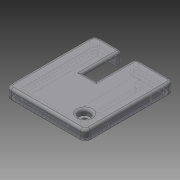
# Autodesk Inventor part: CaseTop_V3
Saved by Autodesk Inventor 2015 SP2 (Build 190223200, 223)
## iProperties
Created: 2016-03-02
Part Number: CaseTop_V3
Material: Generic
Document SubType Name: Modeling
Designer: Iain
Density: 1 g/cm^3
Appearance: Default
Author: Iain
Autodesk Inventor part; units mm, degrees
ref_plane "YZ Plane" through (0, 0, 0) normal (1, 0, 0) x (0, 1, 0)
ref_plane "XZ Plane" through (0, 0, 0) normal (0, 1, 0) x (-1, 0, 0)
ref_plane "XY Plane" through (0, 0, 0) normal (0, 0, 1) x (1, 0, 0)
sketch "Sketch1" plane through (0, 0, 0) normal (0, 0, 1) x (1, 0, 0)
  line L0 (20.25, -0.0291) -> (-20.25, -0.0291) construction
  arc A0 (-20.25, -0.0291) -> (-36.25, -16.0291) centre (-20.25, -16.0291) ccw construction
  line L1 (-36.25, -16.0291) -> (-36.25, -62.0291) construction
  arc A1 (-36.25, -62.0291) -> (-20.25, -78.0291) centre (-20.25, -62.0291) ccw construction
  line L2 (-20.25, -78.0291) -> (20.25, -78.0291) construction
  arc A2 (20.25, -78.0291) -> (36.25, -62.0291) centre (20.25, -62.0291) ccw construction
  line L3 (36.25, -62.0291) -> (36.25, -16.0291) construction
  arc A3 (36.25, -16.0291) -> (20.25, -0.0291) centre (20.25, -16.0291) ccw construction
  circle A4 centre (-34.25, -18.0291) radius 0.5 construction
  circle A5 centre (-34.25, -24.0291) radius 0.5 construction
  circle A6 centre (-34.25, -30.0291) radius 0.5 construction
  circle A7 centre (-34.25, -36.0291) radius 0.5 construction
  circle A8 centre (-34.25, -57.0291) radius 0.5 construction
  circle A9 centre (-34.25, -51.0291) radius 0.5 construction
  circle A10 centre (-34.25, -45.0291) radius 0.5 construction
  circle A11 centre (-34.25, -39.0291) radius 0.5 construction
  circle A12 centre (-34.25, -42.0291) radius 0.5 construction
  circle A13 centre (-34.25, -48.0291) radius 0.5 construction
  circle A14 centre (-34.25, -54.0291) radius 0.5 construction
  circle A15 centre (-34.25, -60.0291) radius 0.5 construction
  circle A16 centre (-34.25, -33.0291) radius 0.5 construction
  circle A17 centre (-34.25, -27.0291) radius 0.5 construction
  circle A18 centre (-34.25, -21.0291) radius 0.5 construction
  circle A19 centre (34.25, -27.0291) radius 0.5 construction
  circle A20 centre (34.25, -33.0291) radius 0.5 construction
  circle A21 centre (34.25, -60.0291) radius 0.5 construction
  circle A22 centre (34.25, -54.0291) radius 0.5 construction
  circle A23 centre (34.25, -48.0291) radius 0.5 construction
  circle A24 centre (34.25, -42.0291) radius 0.5 construction
  circle A25 centre (34.25, -39.0291) radius 0.5 construction
  circle A26 centre (34.25, -45.0291) radius 0.5 construction
  circle A27 centre (34.25, -51.0291) radius 0.5 construction
  circle A28 centre (34.25, -57.0291) radius 0.5 construction
  circle A29 centre (34.25, -36.0291) radius 0.5 construction
  circle A30 centre (34.25, -30.0291) radius 0.5 construction
  circle A31 centre (34.25, -24.0291) radius 0.5 construction
  circle A32 centre (34.25, -18.0291) radius 0.5 construction
  circle A33 centre (34.25, -21.0291) radius 0.5 construction
  circle A34 centre (-18, -76.0291) radius 0.5 construction
  circle A35 centre (-12, -76.0291) radius 0.5 construction
  circle A36 centre (-6, -76.0291) radius 0.5 construction
  circle A37 centre (18, -76.0291) radius 0.5 construction
  circle A38 centre (12, -76.0291) radius 0.5 construction
  circle A39 centre (6, -76.0291) radius 0.5 construction
  circle A40 centre (0, -76.0291) radius 0.5 construction
  circle A41 centre (3, -76.0291) radius 0.5 construction
  circle A42 centre (9, -76.0291) radius 0.5 construction
  circle A43 centre (15, -76.0291) radius 0.5 construction
  circle A44 centre (-3, -76.0291) radius 0.5 construction
  circle A45 centre (-9, -76.0291) radius 0.5 construction
  circle A46 centre (-15, -76.0291) radius 0.5 construction
  circle A47 centre (-9, -2.0291) radius 0.5 construction
  circle A48 centre (-3, -2.0291) radius 0.5 construction
  circle A49 centre (15, -2.0291) radius 0.5 construction
  circle A50 centre (9, -2.0291) radius 0.5 construction
  circle A51 centre (3, -2.0291) radius 0.5 construction
  circle A52 centre (0, -2.0291) radius 0.5 construction
  circle A53 centre (6, -2.0291) radius 0.5 construction
  circle A54 centre (12, -2.0291) radius 0.5 construction
  circle A55 centre (18, -2.0291) radius 0.5 construction
  circle A56 centre (-6, -2.0291) radius 0.5 construction
  circle A57 centre (-12, -2.0291) radius 0.5 construction
  circle A58 centre (-18, -2.0291) radius 0.5 construction
  circle A59 centre (-15, -2.0291) radius 0.5 construction
  arc A60 (-24.75, -62.0291) -> (-20.25, -66.5291) centre (-20.25, -62.0291) ccw construction
  line L4 (-24.75, -16.0291) -> (-24.75, -62.0291) construction
  arc A61 (-20.25, -11.5291) -> (-24.75, -16.0291) centre (-20.25, -16.0291) ccw construction
  line L5 (20.25, -11.5291) -> (-20.25, -11.5291) construction
  arc A62 (24.75, -16.0291) -> (20.25, -11.5291) centre (20.25, -16.0291) ccw construction
  line L6 (24.75, -62.0291) -> (24.75, -16.0291) construction
  arc A63 (20.25, -66.5291) -> (24.75, -62.0291) centre (20.25, -62.0291) ccw construction
  line L7 (-20.25, -66.5291) -> (20.25, -66.5291) construction
  line L8 (-20.25, -15.2291) -> (7.75, -15.2291) construction
  arc A64 (-20.25, -15.2291) -> (-21.05, -16.0291) centre (-20.25, -16.0291) ccw construction
  line L9 (-21.05, -62.0291) -> (-21.05, -16.0291) construction
  arc A65 (-21.05, -62.0291) -> (-20.25, -62.8291) centre (-20.25, -62.0291) ccw construction
  line L10 (20.25, -62.8291) -> (-20.25, -62.8291) construction
  arc A66 (20.25, -62.8291) -> (21.05, -62.0291) centre (20.25, -62.0291) ccw construction
  line L11 (21.05, -23.4291) -> (21.05, -62.0291) construction
  line L12 (21.05, -23.4291) -> (20.25, -23.4291) construction
  line L13 (20.25, -23.4291) -> (20.25, -48.5291) projected
  line L14 (20.25, -48.5291) -> (11.35, -48.5291) projected
  line L15 (11.35, -48.5291) -> (11.35, -23.4291) projected
  line L16 (11.35, -23.4291) -> (11.25, -23.4291) construction
  line L17 (11.25, -23.4291) -> (11.25, -19.4291) construction
  line L18 (11.25, -19.4291) -> (10.25, -19.4291) construction
  line L19 (10.25, -48.5291) -> (10.25, -19.4291) construction
  arc A67 (10.25, -48.5291) -> (11.25, -49.5291) centre (11.25, -48.5291) ccw construction
  line L20 (19.45, -49.5291) -> (11.25, -49.5291) construction
  line L21 (19.45, -62.5291) -> (19.45, -49.5291) construction
  line L22 (-20.75, -62.5291) -> (19.45, -62.5291) construction
  line L23 (-20.75, -15.5291) -> (-20.75, -62.5291) construction
  line L24 (7.75, -15.5291) -> (-20.75, -15.5291) construction
  line L25 (7.75, -15.5291) -> (7.75, -15.2291) construction
  line L26 (21.85, -16.0291) -> (21.85, -62.0291) projected
  arc A68 (20.25, -63.6291) -> (21.85, -62.0291) centre (20.25, -62.0291) ccw projected
  line L27 (20.25, -63.6291) -> (-20.25, -63.6291) projected
  arc A69 (-21.85, -62.0291) -> (-20.25, -63.6291) centre (-20.25, -62.0291) ccw projected
  line L28 (-21.85, -62.0291) -> (-21.85, -16.0291) projected
  arc A70 (-20.25, -14.4291) -> (-21.85, -16.0291) centre (-20.25, -16.0291) ccw projected
  line L29 (-20.25, -14.4291) -> (20.25, -14.4291) projected
  arc A71 (21.85, -16.0291) -> (20.25, -14.4291) centre (20.25, -16.0291) ccw projected
  arc A72 (20.25, -65.0291) -> (23.25, -62.0291) centre (20.25, -62.0291) ccw projected
  line L30 (23.25, -62.0291) -> (23.25, -16.0291) projected
  arc A73 (23.25, -16.0291) -> (20.25, -13.0291) centre (20.25, -16.0291) ccw projected
  line L31 (20.25, -13.0291) -> (-20.25, -13.0291) projected
  arc A74 (-20.25, -13.0291) -> (-23.25, -16.0291) centre (-20.25, -16.0291) ccw projected
  line L32 (-23.25, -16.0291) -> (-23.25, -62.0291) projected
  arc A75 (-23.25, -62.0291) -> (-20.25, -65.0291) centre (-20.25, -62.0291) ccw projected
  line L33 (-20.25, -65.0291) -> (20.25, -65.0291) projected
  line L34 (-8.75, -17.5291) -> (-2.25, -17.5291) construction
  arc A76 (-0.75, -16.0291) -> (-2.25, -17.5291) centre (-0.75, -17.5291) ccw construction
  line L35 (-10.25, -16.0291) -> (-0.75, -16.0291) projected
  arc A77 (-8.75, -17.5291) -> (-10.25, -16.0291) centre (-10.25, -17.5291) ccw construction
  line L36 (9.75, -19.4291) -> (7.75, -19.4291) projected
  line L37 (7.75, -19.4291) -> (7.75, -54.5291) construction
  line L38 (7.75, -54.5291) -> (-18.75, -54.5291) construction
  line L39 (-18.75, -54.5291) -> (-18.75, -24.0291) projected
  line L40 (-18.75, -24.0291) -> (-20.25, -24.0291) projected
  line L41 (-20.25, -62.0291) -> (-20.25, -24.0291) projected
  line L42 (18.95, -62.0291) -> (-20.25, -62.0291) projected
  line L43 (18.95, -62.0291) -> (18.95, -50.0291) projected
  line L44 (18.95, -50.0291) -> (11.25, -50.0291) projected
  arc A78 (9.75, -48.5291) -> (11.25, -50.0291) centre (11.25, -48.5291) ccw projected
  line L45 (9.75, -48.5291) -> (9.75, -19.4291) projected
  circle A79 centre (13.85, -56.0291) radius 1.6 projected
  line L46 (7.75, -15.9291) -> (7.75, -17.5291) construction
  line L47 (-0.75, -17.5291) -> (7.75, -17.5291) construction
  line L48 (-0.75, -19.0291) -> (-0.75, -17.5291) construction
  line L49 (-10.25, -19.0291) -> (-0.75, -19.0291) construction
  line L50 (-10.25, -17.5291) -> (-10.25, -19.0291) construction
  line L51 (-18.75, -17.5291) -> (-10.25, -17.5291) construction
  line L52 (-18.75, -24.0291) -> (-18.75, -17.5291) construction
  line L53 (-18.75, -24.0291) -> (-18.75, -54.5291) construction
  line L54 (-18.75, -54.5291) -> (7.75, -54.5291) projected
  line L55 (7.75, -54.5291) -> (7.75, -17.9291) projected
  line L56 (12.75, -17.9291) -> (7.75, -17.9291) construction
  line L57 (12.75, -21.9291) -> (12.75, -17.9291) construction
  line L58 (13.05, -21.9291) -> (12.75, -21.9291) construction
  line L59 (13.05, -16.9291) -> (13.05, -21.9291) construction
  line L60 (18.55, -16.9291) -> (13.05, -16.9291) construction
  line L61 (18.55, -21.9291) -> (18.55, -16.9291) construction
  line L62 (20.35, -21.9291) -> (18.55, -21.9291) construction
  line L63 (20.35, -15.9291) -> (20.35, -21.9291) construction
  line L64 (7.75, -15.9291) -> (20.35, -15.9291) construction
  line L65 (20.25, -23.4291) -> (18.55, -23.4291) construction
  line L66 (13.05, -23.4291) -> (11.35, -23.4291) construction
  line L67 (-10.25, -16.0291) -> (-20.25, -16.0291)
  line L68 (-20.25, -16.0291) -> (-20.25, -24.0291)
  line L69 (7.75, -14.4291) -> (7.75, -16.0291)
  point P0 (0, 0)
  point P1 (0, -14.4291)
  point P2 (-0.75, 31.777)
  point P3 (-0.75, 19.2242)
  point P4 (-0.75, 27.5206)
  constraints: 6 end point, 2 horizontal alignment, 2 parallel, 1 midpoint, 1 tangent, 1 vertical, 1 vertical alignment
sketch "Sketch2" plane through (0, 0, 0) normal (0, 0, 1) x (1, 0, 0)
  line L0 (20.25, -13.0291) -> (-20.25, -13.0291) projected
  arc A0 (-20.25, -13.0291) -> (-23.25, -16.0291) centre (-20.25, -16.0291) ccw projected
  line L1 (-23.25, -16.0291) -> (-23.25, -62.0291) projected
  arc A1 (-23.25, -62.0291) -> (-20.25, -65.0291) centre (-20.25, -62.0291) ccw projected
  line L2 (-20.25, -65.0291) -> (20.25, -65.0291) projected
  arc A2 (20.25, -65.0291) -> (23.25, -62.0291) centre (20.25, -62.0291) ccw projected
  line L3 (23.25, -62.0291) -> (23.25, -16.0291) projected
  arc A3 (23.25, -16.0291) -> (20.25, -13.0291) centre (20.25, -16.0291) ccw projected
  point P0 (0, 0)
extrude "Extrusion1" add sketch "Sketch2" against normal blind 1.5
sketch "Sketch3" plane through (0, 0, -1.5) normal (0, 0, -1) x (1, 0, 0)
  line L0 (-20.25, 13.0291) -> (20.25, 13.0291) projected
  arc A0 (-23.25, 16.0291) -> (-20.25, 13.0291) centre (-20.25, 16.0291) ccw projected
  line L1 (-23.25, 62.0291) -> (-23.25, 16.0291) projected
  arc A1 (-20.25, 65.0291) -> (-23.25, 62.0291) centre (-20.25, 62.0291) ccw projected
  line L2 (20.25, 65.0291) -> (-20.25, 65.0291) projected
  arc A2 (23.25, 62.0291) -> (20.25, 65.0291) centre (20.25, 62.0291) ccw projected
  line L3 (23.25, 16.0291) -> (23.25, 62.0291) projected
  arc A3 (20.25, 13.0291) -> (23.25, 16.0291) centre (20.25, 16.0291) ccw projected
  arc A4 (-21.75, 16.0291) -> (-20.25, 14.5291) centre (-20.25, 16.0291) ccw
  line L4 (-20.25, 14.5291) -> (20.25, 14.5291)
  arc A5 (20.25, 14.5291) -> (21.75, 16.0291) centre (20.25, 16.0291) ccw
  line L5 (21.75, 16.0291) -> (21.75, 62.0291)
  arc A6 (21.75, 62.0291) -> (20.25, 63.5291) centre (20.25, 62.0291) ccw
  line L6 (20.25, 63.5291) -> (-20.25, 63.5291)
  arc A7 (-20.25, 63.5291) -> (-21.75, 62.0291) centre (-20.25, 62.0291) ccw
  line L7 (-21.75, 62.0291) -> (-21.75, 16.0291)
  dimension "d13" = 1.5
  constraints: 8 end point, 8 point on circle, 4 centre point, 7 other
  measures "d13" distance between parallel lines of L1 L7
extrude "Extrusion2" add sketch "Sketch3" along normal blind 4.1
sketch "Sketch5" plane through (0, 0, -1.5) normal (0, 0, -1) x (-1, 0, 0)
  line L0 (21.75, -62.0291) -> (21.75, -16.0291) projected
  arc A0 (21.75, -16.0291) -> (20.25, -14.5291) centre (20.25, -16.0291) ccw projected
  line L1 (20.25, -14.5291) -> (-20.25, -14.5291) projected
  arc A1 (-20.25, -14.5291) -> (-21.75, -16.0291) centre (-20.25, -16.0291) ccw projected
  line L2 (-21.75, -16.0291) -> (-21.75, -62.0291) projected
  arc A2 (-21.75, -62.0291) -> (-20.25, -63.5291) centre (-20.25, -62.0291) ccw projected
  line L3 (-20.25, -63.5291) -> (20.25, -63.5291) projected
  arc A3 (20.25, -63.5291) -> (21.75, -62.0291) centre (20.25, -62.0291) ccw projected
  line L4 (-18.75, -60.5291) -> (-18.75, -51.5291)
  line L5 (-18.75, -17.5291) -> (-8.25, -17.5291) construction
  line L6 (18.75, -17.5291) -> (18.75, -60.5291)
  line L7 (18.75, -60.5291) -> (-18.75, -60.5291)
  line L8 (-18.95, -50.0291) -> (-11.25, -50.0291) projected
  line L9 (-9.75, -48.5291) -> (-9.75, -19.4291) projected
  line L10 (-7.75, -15.9291) -> (-7.75, -17.5291) construction
  line L11 (-18.75, -51.5291) -> (-8.25, -51.5291)
  line L12 (-8.25, -17.5291) -> (-8.25, -51.5291)
  line L13 (-18.75, -51.5291) -> (-18.75, -17.5291) construction
  line L14 (-8.25, -17.5291) -> (18.75, -17.5291)
  point P0 (0, 0)
  dimension "d14" = 3
  dimension "d15" = 1.5
  dimension "d16" = 1.5
  dimension "d17" = 3
  dimension "d18" = 3
  dimension "d19" = 34
  dimension "d20" = 10.5
  constraints: 16 end point, 1 horizontal, 1 vertical, 1 other
  measures "d14" distance between parallel lines of L2 L4
  measures "d15" distance between parallel lines of L11 L8
  measures "d16" distance between parallel lines of L9 L12
  measures "d17" distance between parallel lines of L1 L14
  measures "d18" distance between parallel lines of L0 L6
  measures "d19" distance of L4.end L5.start
  measures "d20" distance of L5.start L5.end
extrude "Extrusion4" add sketch "Sketch5" along normal blind 5.6
ref_plane "Work Plane1" through (11.35, -48.5291, 0) normal (0, 1, 0) x (1, 0, 0)
sketch "Sketch6" plane through (11.35, -48.5291, 0) normal (0, 1, 0) x (1, 0, 0)
  line L0 (8.9, 0) -> (0, 0) projected
  line L1 (7.4, 7.1) -> (-3.1, 7.1) projected
  circle A0 centre (4.45, 7.1) radius 4.45
  point P0 (-11.35, 0)
  point P1 (4.45, 0)
  point P2 (2.15, 7.1)
  dimension "d27" = 8.9
  constraints: 2 midpoint, 1 centre point, 1 horizontal alignment, 1 vertical alignment
  measures "d27" diameter of A0
extrude "Extrusion5" cut sketch "Sketch6" along normal blind 25.1
sketch "Sketch7" plane through (0, 0, -7.1) normal (0, 0, -1) x (-1, 0, 0)
  line L0 (-20.25, -48.5291) -> (-20.25, -23.4291) projected
  line L1 (-20.25, -23.4291) -> (-11.35, -23.4291) projected
  line L2 (-11.35, -23.4291) -> (-11.35, -48.5291) projected
  line L3 (-11.35, -48.5291) -> (-20.25, -48.5291) projected
  line L4 (18.75, -60.5291) -> (-18.75, -60.5291) projected
  line L5 (-18.75, -60.5291) -> (-18.75, -51.5291) projected
  line L6 (-18.75, -51.5291) -> (-8.25, -51.5291) projected
  line L7 (-8.25, -51.5291) -> (-8.25, -17.5291) projected
  line L8 (-8.25, -17.5291) -> (18.75, -17.5291) projected
  line L9 (18.75, -17.5291) -> (18.75, -60.5291) projected
  line L10 (21.75, -62.0291) -> (21.75, -16.0291) projected
  arc A0 (21.75, -16.0291) -> (20.25, -14.5291) centre (20.25, -16.0291) ccw projected
  line L11 (20.25, -14.5291) -> (-20.25, -14.5291) projected
  arc A1 (-20.25, -14.5291) -> (-21.75, -16.0291) centre (-20.25, -16.0291) ccw projected
  line L12 (-21.75, -16.0291) -> (-21.75, -62.0291) projected
  arc A2 (-21.75, -62.0291) -> (-20.25, -63.5291) centre (-20.25, -62.0291) ccw projected
  line L13 (-20.25, -63.5291) -> (20.25, -63.5291) projected
  arc A3 (20.25, -63.5291) -> (21.75, -62.0291) centre (20.25, -62.0291) ccw projected
  line L14 (-20.25, -62.0291) -> (-20.25, -16.0291) construction
  line L15 (-20.25, -16.0291) -> (20.25, -16.0291) construction
  line L16 (20.25, -16.0291) -> (20.25, -62.0291) construction
  line L17 (20.25, -62.0291) -> (-20.25, -62.0291) construction
  line L18 (-20.25, -23.4291) -> (-11.35, -23.4291) construction
  line L19 (-20.25, -16.0291) -> (-11.35, -16.0291)
  line L20 (-11.35, -16.0291) -> (-11.35, -23.4291)
  line L21 (-11.35, -23.4291) -> (-20.25, -23.4291)
  line L22 (-20.25, -23.4291) -> (-20.25, -16.0291)
  line L23 (-11.35, -16.0291) -> (18.75, -16.0291)
  line L24 (18.75, -16.0291) -> (18.75, -17.5291)
  line L25 (18.75, -17.5291) -> (-11.35, -17.5291)
  line L26 (-11.35, -17.5291) -> (-11.35, -16.0291)
  line L27 (8.75, -17.5291) -> (2.25, -17.5291) construction
  line L28 (2.25, -16.0291) -> (8.75, -16.0291)
  line L29 (8.75, -16.0291) -> (8.75, -17.5291)
  line L30 (8.75, -17.5291) -> (2.25, -17.5291)
  line L31 (2.25, -17.5291) -> (2.25, -16.0291)
  line L32 (-11.35, -16.0291) -> (-8.25, -16.0291)
  line L33 (-8.25, -16.0291) -> (-8.25, -21.0291)
  line L34 (-8.25, -21.0291) -> (-11.35, -21.0291)
  line L35 (-11.35, -21.0291) -> (-11.35, -16.0291)
  point P0 (0, 0)
  point P1 (-15.8, -16.0291)
  point P2 (-15.8, -23.4291)
  point P3 (-15.8, -23.4291)
  point P4 (-20.25, -19.7291)
  point P5 (-11.35, -19.7291)
  point P6 (3.7, -16.0291)
  point P7 (3.7, -17.5291)
  point P8 (5.25, -17.5291)
  point P9 (-11.35, -16.7791)
  point P10 (18.75, -16.7791)
  point P11 (8.75, -16.7791)
  point P12 (2.25, -16.7791)
  point P13 (5.5, -16.0291)
  point P14 (5.5, -17.5291)
  point P15 (-11.35, -18.5291)
  point P16 (-8.25, -18.5291)
  point P17 (-9.8, -16.0291)
  dimension "d28" = 1.5
  dimension "d31" = 5
  constraints: 40 end point, 17 midpoint, 8 parallel, 8 vertical alignment, 6 horizontal alignment, 4 horizontal, 4 perpendicular, 1 coincident, 3 other
  measures "d28" distance between parallel lines of L12 L14
  measures "d31" distance of L32.end L33.end
extrude "Extrusion6" cut sketch "Sketch7" against normal up to surface (5.6 mm away) contours L22 L19 L20 L1 | L20 L25 L7 L34 | L23 L33 L25 L20 | L23 L31 L8 L33 | L23 L29 L8 L31 | L23 L24 L8 L29
sketch "Sketch8" plane through (0, 0, -1.5) normal (0, 0, -1) x (-1, 0, 0)
  line L0 (21.75, -62.0291) -> (21.75, -16.0291) projected
  arc A0 (21.75, -16.0291) -> (20.25, -14.5291) centre (20.25, -16.0291) ccw projected
  line L1 (20.25, -14.5291) -> (-20.25, -14.5291) projected
  arc A1 (-20.25, -14.5291) -> (-21.75, -16.0291) centre (-20.25, -16.0291) ccw projected
  line L2 (-21.75, -16.0291) -> (-21.75, -62.0291) projected
  arc A2 (-21.75, -62.0291) -> (-20.25, -63.5291) centre (-20.25, -62.0291) ccw projected
  line L3 (-20.25, -63.5291) -> (20.25, -63.5291) projected
  arc A3 (20.25, -63.5291) -> (21.75, -62.0291) centre (20.25, -62.0291) ccw projected
  line L4 (-20.25, -23.4291) -> (-20.25, -16.0291) projected
  line L5 (-20.25, -16.0291) -> (18.75, -16.0291) projected
  line L6 (18.75, -16.0291) -> (18.75, -60.5291) projected
  line L7 (18.75, -60.5291) -> (-18.75, -60.5291) projected
  line L8 (-18.75, -60.5291) -> (-18.75, -51.5291) projected
  line L9 (-18.75, -51.5291) -> (-8.25, -51.5291) projected
  line L10 (-8.25, -51.5291) -> (-8.25, -21.0291) projected
  line L11 (-8.25, -21.0291) -> (-11.35, -21.0291) projected
  line L12 (-11.35, -21.0291) -> (-11.35, -23.4291) projected
  line L13 (-11.35, -23.4291) -> (-11.35, -48.5291) projected
  line L14 (-11.35, -48.5291) -> (-20.25, -48.5291) projected
  line L15 (-20.25, -48.5291) -> (-20.25, -23.4291) projected
  line L16 (-18.75, -51.5291) -> (-8.25, -51.5291)
  line L17 (-8.25, -51.5291) -> (-8.25, -60.5291)
  line L18 (-8.25, -60.5291) -> (-18.75, -60.5291)
  line L19 (-18.75, -60.5291) -> (-18.75, -51.5291)
  line L20 (-18.75, -60.5291) -> (-18.75, -51.5291) projected
  point P0 (0, 0)
  point P1 (-18.75, -56.0291)
  point P2 (-18.75, -56.0291)
  point P3 (-8.25, -56.0291)
  point P4 (-13.5, -60.5291)
  point P5 (-13.5, -51.5291)
  constraints: 8 end point, 5 midpoint, 2 horizontal alignment, 2 parallel, 1 coincident, 1 horizontal, 1 perpendicular, 1 vertical alignment
extrude "Extrusion7" add sketch "Sketch8" along normal up to surface (5.6 mm away) contours L7 L8 L9 L17
sketch "Sketch10" plane through (0, 0, 0) normal (0, 0, 1) x (1, 0, 0)
  circle A0 centre (13.85, -56.0291) radius 1.6 projected
  point P0 (0, 0)
  constraints: 1 coincident
hole "Hole1" at (13.85, -56.0291, 0) direction (0, 0, -1) diameter 3.2 end through all
sketch "Sketch11" plane through (0, 0, 0) normal (0, 0, 1) x (1, 0, 0)
  circle A0 centre (13.85, -56.0291) radius 1.6 projected
  line L0 (20.25, -13.0291) -> (-20.25, -13.0291) projected
  arc A1 (-20.25, -13.0291) -> (-23.25, -16.0291) centre (-20.25, -16.0291) ccw projected
  line L1 (-23.25, -16.0291) -> (-23.25, -62.0291) projected
  arc A2 (-23.25, -62.0291) -> (-20.25, -65.0291) centre (-20.25, -62.0291) ccw projected
  line L2 (-20.25, -65.0291) -> (20.25, -65.0291) projected
  arc A3 (20.25, -65.0291) -> (23.25, -62.0291) centre (20.25, -62.0291) ccw projected
  line L3 (23.25, -62.0291) -> (23.25, -16.0291) projected
  arc A4 (23.25, -16.0291) -> (20.25, -13.0291) centre (20.25, -16.0291) ccw projected
  circle A5 centre (13.85, -56.0291) radius 3.15
  point P0 (0, 0)
  dimension "d49" = 6.3
  constraints: 1 centre point, 1 coincident
  measures "d49" diameter of A5
extrude "Extrusion9" cut sketch "Sketch11" against normal blind 3.4 contours A5
fillet "OverlapRimFillet" radius 0.8 8 edges at (21.3107, -14.9685, -7.1) (21.75, -39.0291, -7.1) (21.3107, -63.0898, -7.1) (0, -63.5291, -7.1) (-21.3107, -63.0898, -7.1) (-21.75, -39.0291, -7.1) (-21.3107, -14.9685, -7.1) (0, -14.5291, -7.1)
sketch "Sketch9" plane through (0, 0, -7.1) normal (0, 0, -1) x (-1, 0, 0)
  line L0 (7.25, -36.0291) -> (-0.75, -36.0291)
  line L1 (-0.75, -36.0291) -> (-0.75, -13.0291)
  line L2 (-0.75, -13.0291) -> (7.25, -13.0291)
  line L3 (7.25, -13.0291) -> (7.25, -36.0291)
  line L4 (21.75, -16.0291) -> (21.75, -62.0291) projected
  arc A0 (20.25, -63.5291) -> (21.75, -62.0291) centre (20.25, -62.0291) ccw projected
  line L5 (20.25, -63.5291) -> (-20.25, -63.5291) projected
  arc A1 (-21.75, -62.0291) -> (-20.25, -63.5291) centre (-20.25, -62.0291) ccw projected
  line L6 (-21.75, -62.0291) -> (-21.75, -16.0291) projected
  arc A2 (-20.25, -14.5291) -> (-21.75, -16.0291) centre (-20.25, -16.0291) ccw projected
  line L7 (-20.25, -14.5291) -> (20.25, -14.5291) projected
  arc A3 (21.75, -16.0291) -> (20.25, -14.5291) centre (20.25, -16.0291) ccw projected
  line L8 (20.25, -13.0291) -> (-20.25, -13.0291) projected
  arc A4 (-20.25, -13.0291) -> (-23.25, -16.0291) centre (-20.25, -16.0291) ccw projected
  line L9 (-23.25, -16.0291) -> (-23.25, -62.0291) projected
  arc A5 (-23.25, -62.0291) -> (-20.25, -65.0291) centre (-20.25, -62.0291) ccw projected
  line L10 (-20.25, -65.0291) -> (20.25, -65.0291) projected
  arc A6 (20.25, -65.0291) -> (23.25, -62.0291) centre (20.25, -62.0291) ccw projected
  line L11 (23.25, -62.0291) -> (23.25, -16.0291) projected
  arc A7 (23.25, -16.0291) -> (20.25, -13.0291) centre (20.25, -16.0291) ccw projected
  line L12 (-9.75, -48.5291) -> (-9.75, -19.4291) projected
  line L13 (-20.25, -16.0291) -> (18.75, -16.0291) projected
  point P0 (0, 0)
  point P1 (3.25, -13.0291)
  point P2 (0, -14.5291)
  point P3 (0, -13.0291)
  dimension "d36" = 8
  dimension "d37" = 9
  dimension "d38" = 20
  constraints: 8 end point, 3 midpoint, 2 parallel, 1 horizontal, 1 horizontal alignment, 1 perpendicular
  measures "d36" distance of L0.start L0.end
  measures "d37" distance from line of L0.end L12
  measures "d38" distance between parallel lines of L13 L0
extrude "LEDSlot" cut sketch "Sketch9" against normal through all contours L0 L1 L13 L3 | L13 L1 L7 L3 | L7 L1 L2 L3
fillet "SlotFillet" radius 1.5 14 edges at (22.3713, -13.9078, 0) (23.25, -39.0291, 0) (22.3713, -64.1505, 0) (0, -65.0291, 0) (-22.3713, -64.1505, 0) (-23.25, -39.0291, 0) (-22.3713, -13.9078, 0) (-13.75, -13.0291, 0) (10.5, -13.0291, 0) (0.75, -24.5291, 0) (-7.25, -24.5291, 0) (-3.25, -36.0291, 0) (0.75, -13.0291, -2.8) (-7.25, -13.0291, -2.8)
fillet "Fillet3" radius 1.5 1 edges at (10.7, -56.0291, 0)
equation "\"d13\" = minWallThickness"
equation "\"d17\" = d14"
equation "\"d18\" = d14"
equation "\"minWallThickness\" = 1.5"
body "Solid1"
